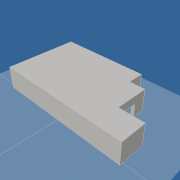
# Autodesk Inventor part: Basis
Saved by Autodesk Inventor 2016 SP2 (Build 200236200, 236)
## iProperties
Created: 2018-07-08
Part Number: Basis
Material: Generisch
Document SubType Name: Modeling
Designer: User
Density: 1 g/cm^3
Appearance: Vorgabe
Author: User
Autodesk Inventor part; units mm, degrees
ref_plane "YZ Plane" through (0, 0, 0) normal (1, 0, 0) x (0, 1, 0)
ref_plane "XZ Plane" through (0, 0, 0) normal (0, 1, 0) x (-1, 0, 0)
ref_plane "XY Plane" through (0, 0, 0) normal (0, 0, 1) x (1, 0, 0)
sketch "Skizze1" plane through (0, 0, 0) normal (0, 0, 1) x (1, 0, 0)
  line L0 (-65, 0) -> (65, 0)
  line L1 (65, 0) -> (65, 20)
  line L2 (65, 20) -> (40, 20)
  line L3 (40, 20) -> (40, 54)
  line L4 (-65, 41) -> (-65, 0)
  line L5 (-65, 41) -> (-65, 41)
  line L6 (-65, 54) -> (-65, 54)
  line L7 (-65, 54) -> (-65, 41)
  line L8 (24, 71) -> (24, 54)
  line L9 (24, 54) -> (40, 54)
  circle A0 centre (-59.5, 2.832) radius 1.25
  circle A1 centre (23.1262, 2.832) radius 1.25
  circle A2 centre (23.1262, 51.168) radius 1.25
  circle A3 centre (-52.007, 51.168) radius 1.25
  line L10 (25.8762, 2.832) -> (25.8762, 0)
  line L11 (25.8762, 0) -> (20.3762, 0)
  line L12 (20.3762, 0) -> (20.3762, 2.832)
  arc A4 (25.8762, 2.832) -> (20.3762, 2.832) centre (23.1262, 2.832) ccw
  line L13 (-56.75, 0) -> (-56.75, 2.832)
  line L14 (-62.25, 0) -> (-62.25, 2.832)
  line L15 (-56.75, 0) -> (-62.25, 0)
  arc A5 (-56.75, 2.832) -> (-62.25, 2.832) centre (-59.5, 2.832) ccw
  line L16 (25.8762, 51.168) -> (25.8762, 54)
  line L17 (25.8762, 54) -> (20.3762, 54)
  line L18 (20.3762, 54) -> (20.3762, 51.168)
  arc A6 (20.3762, 51.168) -> (25.8762, 51.168) centre (23.1262, 51.168) ccw
  line L19 (-49.257, 51.168) -> (-49.257, 54)
  line L20 (-49.257, 54) -> (-54.757, 54)
  line L21 (-54.757, 54) -> (-54.757, 51.168)
  arc A7 (-54.757, 51.168) -> (-49.257, 51.168) centre (-52.007, 51.168) ccw
  line L22 (-65, 54) -> (24, 54)
  line L23 (24, 54) -> (24, 57)
  line L24 (24, 57) -> (-65, 57)
  line L25 (-65, 57) -> (-65, 54)
  line L26 (24, 71) -> (-65, 71)
  line L27 (-65, 71) -> (-65, 54)
  line L28 (43, 23) -> (68, 23)
  line L29 (68, 23) -> (68, -3)
  line L30 (68, -3) -> (-68, -3)
  line L31 (-68, -3) -> (-68, 44)
  line L32 (-68, 44) -> (-68, 44)
  line L33 (-68, 44) -> (-68, 57)
  line L34 (-68, 57) -> (-68, 57)
  line L35 (-68, 57) -> (-68, 74)
  line L36 (-68, 74) -> (27, 74)
  line L37 (27, 74) -> (27, 57)
  line L38 (27, 57) -> (43, 57)
  line L39 (43, 57) -> (43, 23)
  line L40 (-65, 71) -> (-51, 71)
  line L41 (-51, 71) -> (-51, 66)
  line L42 (-51, 66) -> (-65, 66)
  line L43 (-65, 66) -> (-65, 71)
  line L44 (8, 71) -> (-8, 71)
  line L45 (-8, 71) -> (-8, 66)
  line L46 (-8, 66) -> (8, 66)
  line L47 (8, 66) -> (8, 71)
  line L48 (-65, 71) -> (-55, 71)
  line L49 (-55, 71) -> (-55, 66)
  line L50 (-55, 66) -> (-65, 66)
  line L51 (-65, 66) -> (-65, 71)
  line L52 (1, 71) -> (-4, 71)
  line L53 (-4, 71) -> (-4, 66)
  line L54 (-4, 66) -> (1, 66)
  line L55 (1, 66) -> (1, 71)
  line L56 (8, 71) -> (1, 71)
  line L57 (1, 71) -> (1, 66)
  line L58 (1, 66) -> (8, 66)
  line L59 (8, 66) -> (8, 71)
  line L60 (-4, 71) -> (-8, 71)
  line L61 (-8, 71) -> (-8, 66)
  line L62 (-8, 66) -> (-4, 66)
  line L63 (-4, 66) -> (-4, 71)
  line L64 (8, 57) -> (-8, 57)
  line L65 (-8, 57) -> (-8, 60.5)
  line L66 (-8, 60.5) -> (8, 60.5)
  line L67 (8, 60.5) -> (8, 57)
  line L68 (1, 60.5) -> (-4, 60.5)
  line L69 (-4, 60.5) -> (-4, 57)
  line L70 (-4, 57) -> (1, 57)
  line L71 (1, 57) -> (1, 60.5)
  line L72 (-65, 57) -> (-51, 57)
  line L73 (-51, 57) -> (-51, 60.5)
  line L74 (-51, 60.5) -> (-65, 60.5)
  line L75 (-65, 60.5) -> (-65, 57)
  line L76 (-55, 60.5) -> (-65, 60.5)
  line L77 (-65, 60.5) -> (-65, 57)
  line L78 (-65, 57) -> (-55, 57)
  line L79 (-55, 57) -> (-55, 60.5)
  point P0 (0, 0)
  point P1 (0, 0)
  point P2 (0, 0)
  dimension "d0" = 130
  dimension "d1" = 25
  dimension "d8" = 20
  dimension "d9" = 41
  dimension "d11" = 54
  dimension "d42" = 5.5
  dimension "d43" = 82.6262
  dimension "d44" = 2.5
  dimension "d45" = 2.832
  dimension "d46" = 7.493
  dimension "d47" = 48.336
  dimension "d48" = 5.5
  dimension "d49" = 5.5
  dimension "d50" = 5.5
  dimension "d51" = 5.5
  dimension "d52" = 3
  dimension "d57" = 0
  dimension "d58" = 89
  dimension "d59" = 71
  dimension "d60" = 3
  dimension "d61" = 2.832
  dimension "d70" = 16
  dimension "d71" = 14
  dimension "d72" = 5
  dimension "d73" = 43
  dimension "d76" = 10
  dimension "d79" = 51
  dimension "d80" = 5
  dimension "d83" = 5.5
  dimension "d84" = 0
  constraints: 161 end point, 26 perpendicular, 22 parallel, 16 horizontal, 14 point on line, 11 collinear, 8 centre point, 8 point on circle, 8 tangent, 6 coincident, 6 vertical, 3 equal radius, 3 horizontal alignment, 1 midpoint, 1 vertical alignment, 11 other
  measures "d0" distance between parallel lines of L1 L4
  measures "d1" distance between parallel lines of L1 L3
  measures "d8" distance between parallel lines of L0 L2
  measures "d9" distance between parallel lines of L0 L5
  measures "d11" distance between parallel lines of L0 L6
  measures "d42" distance from line of L4 A0.centre
  measures "d43" distance of A0.centre A1.centre
  measures "d44" diameter of A0
  measures "d45" distance from line of L0 A0.centre
  measures "d46" horizontal distance of A0.centre A3.centre
  measures "d47" vertical distance of A0.centre A3.centre
  measures "d48" distance between parallel lines of L12 L10
  measures "d49" distance between parallel lines of L14 L13
  measures "d50" distance between parallel lines of L18 L16
  measures "d51" distance between parallel lines of L21 L19
  measures "d52" distance between parallel lines of L22 L24
  measures "d57" distance between parallel lines of L7 L4
  measures "d58" distance of L8.start L26.end
  measures "d59" distance between parallel lines of L0 L26
  measures "d60" distance between parallel lines of L2 L28
  measures "d61" distance from line of L22 A2.centre
  measures "d70" distance of L45.end L46.end
  measures "d71" distance of L41.end L42.end
  measures "d72" distance of L46.end L44.start
  measures "d73" distance between parallel lines of L41 L45
  measures "d76" distance between parallel lines of L27 L49
  measures "d79" distance between parallel lines of L49 L53
  measures "d80" distance between parallel lines of L53 L55
  measures "d83" distance between parallel lines of L66 L58
  measures "d84" distance between parallel lines of L33 L35
extrude "Extrusion1" add sketch "Skizze1" along normal blind 3 contours L4 L7 L22 L21 A7 L19 L18 A6 L16 L9 L3 L2 L1 L0 L10 A4 L12 L13 A5 L14 | L14 A5 L13 L0 | L25 L24 L8 L17 L22 L20 | L12 A4 L10 L0 | L20 L19 A7 L21 | L27 L74 L79 L24 | L79 L74 L73 L24 | L27 L42 L41 L26 L45 L46 L47 L8 L24 L67 L66 L65 L73 L74 | L17 L9 L16 A6 L18 | L27 L26 L49 L42 | L65 L66 L69 L24 | L49 L26 L41 L42 | L69 L66 L71 L24 | L24 L71 L66 L67 | L47 L46 L55 L26 | L26 L53 L46 L45 | L55 L46 L53 L26 | A0 | A1 | A2 | A3 | L28 L29 L30 L31 L33 L35 L36 L37 L38 L39
extrude "Extrusion2" add sketch "Skizze1" against normal blind 20 contours L25 L24 L8 L17 L22 L20 | L27 L26 L49 L42 | L69 L66 L71 L24 | L55 L46 L53 L26 | L28 L29 L30 L31 L33 L35 L36 L37 L38 L39
sketch "Skizze2" plane through (43, 23, 3) normal (1, 0, 0) x (0, 0, -1)
  line L0 (23, 21.75) -> (9, 21.75)
  line L1 (9, 21.75) -> (9, 9.25)
  line L2 (9, 9.25) -> (23, 9.25)
  line L3 (23, 9.25) -> (23, 21.75)
  line L4 (23, 0) -> (0, 0) projected
  line L5 (23, 34) -> (23, 0) projected
  point P0 (3, -23)
  dimension "d62" = 9.25
  dimension "d63" = 21.75
  dimension "d64" = 14
  constraints: 8 end point, 2 parallel, 1 collinear, 1 horizontal, 1 perpendicular
  measures "d62" distance between parallel lines of L4 L2
  measures "d63" distance between parallel lines of L4 L0
  measures "d64" distance between parallel lines of L3 L1
extrude "Extrusion3" cut sketch "Skizze2" against normal up to surface (3 mm away)
extrude "Extrusion6" add sketch "Skizze1" against normal blind 10 contours L27 L74 L79 L24 | L79 L74 L73 L24 | L27 L26 L49 L42 | L65 L66 L69 L24 | L49 L26 L41 L42 | L69 L66 L71 L24 | L24 L71 L66 L67 | L47 L46 L55 L26 | L26 L53 L46 L45 | L55 L46 L53 L26
extrude "Extrusion4" add sketch "Skizze1" against normal blind 4 contours L14 A5 L13 L0 | L12 A4 L10 L0 | L20 L19 A7 L21 | L17 L9 L16 A6 L18
extrude "Extrusion7" cut sketch "Skizze1" along normal blind 1.5 contours A0 | A1 | A2 | A3
sketch "Skizze3" plane through (-68, 74, 3) normal (0, 1, 0) x (1, 0, 0)
  line L0 (0, 0) -> (0, 23) projected
  line L1 (95, 0) -> (0, 0) projected
  line L2 (0, 23) -> (95, 23) projected
  line L3 (13, 13) -> (64, 13)
  line L4 (64, 13) -> (64, 23)
  line L5 (64, 23) -> (13, 23)
  line L6 (13, 23) -> (13, 13)
  point P0 (68, 3)
  dimension "d65" = 13
  dimension "d66" = 13
  dimension "d67" = 51
  constraints: 8 end point, 2 parallel, 1 horizontal, 1 perpendicular, 1 point on line
  measures "d65" distance between parallel lines of L3 L1
  measures "d66" distance between parallel lines of L6 L0
  measures "d67" distance between parallel lines of L4 L6
extrude "Extrusion5" cut sketch "Skizze3" against normal up to surface (3 mm away)
